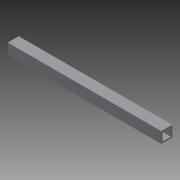
# Autodesk Inventor part: west coast backfront
Saved by Autodesk Inventor 2013 (Build 170138000, 138)
## iProperties
Created: 2014-08-13
Part Number: west coast backfront
Material: Generic
Document SubType Name: Modeling
Designer: kahohbein
Density: 1 g/cm^3
Author: kahohbein
Autodesk Inventor part; units mm, degrees
ref_plane "YZ Plane" through (0, 0, 0) normal (1, 0, 0) x (0, 1, 0)
ref_plane "XZ Plane" through (0, 0, 0) normal (0, 1, 0) x (-1, 0, 0)
ref_plane "XY Plane" through (0, 0, 0) normal (0, 0, 1) x (1, 0, 0)
sketch "Sketch1" plane through (0, 0, 0) normal (0, 0, 1) x (1, 0, 0)
  line L0 (0, 0) -> (355.6, 0)
  line L1 (355.6, 0) -> (355.6, 25.4)
  line L2 (355.6, 25.4) -> (0, 25.4)
  line L3 (0, 25.4) -> (0, 0)
  dimension "d0" = 355.6
  dimension "d1" = 25.4
  constraints: 8 end point, 2 parallel, 1 horizontal, 1 perpendicular
  measures "d0" distance of L2.end L1.end
  measures "d1" distance of L1.end L0.end
extrude "Extrusion1" add sketch "Sketch1" along normal blind 25.4
sketch "Sketch2" plane through (355.6, 0, 0) normal (1, 0, 0) x (0, 0, -1)
  line L0 (-22.225, 3.175) -> (-3.175, 3.175)
  line L1 (-3.175, 3.175) -> (-3.175, 22.225)
  line L2 (-3.175, 22.225) -> (-22.225, 22.225)
  line L3 (-22.225, 22.225) -> (-22.225, 3.175)
  line L4 (-22.225, 3.175) -> (-3.175, 22.225) construction
  line L5 (-3.175, 3.175) -> (-22.225, 22.225) construction
  point P0 (-12.7, 12.7)
  dimension "d4" = 19.05
  dimension "d5" = 19.05
  constraints: 12 end point, 2 midpoint, 2 parallel, 1 horizontal, 1 perpendicular
  measures "d4" distance of L2.end L1.end
  measures "d5" distance of L1.end L0.end
extrude "Extrusion2" cut sketch "Sketch2" against normal blind 355.6
body "Solid1"
